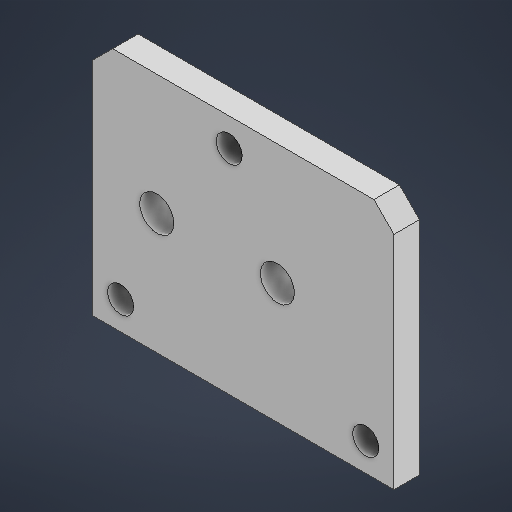
# Autodesk Inventor part: PlacaRedutor
Saved by Autodesk Inventor 2027 (Build 310192060, 192F)
## iProperties
Created: 2026-09-10
Part Number: PlacaRedutor
Material: Genérico
Document SubType Name: Modeling
Designer: Giovanna Oliveira
Density: 1 g/cm^3
Appearance: Padrão
Author: Giovanna Oliveira
Autodesk Inventor part; units mm, degrees
ref_plane "YZ Plane" through (0, 0, 0) normal (1, 0, 0) x (0, 1, 0)
ref_plane "XZ Plane" through (0, 0, 0) normal (0, 1, 0) x (-1, 0, 0)
ref_plane "XY Plane" through (0, 0, 0) normal (0, 0, 1) x (1, 0, 0)
sketch "Esboço5" plane through (0, 0, 0) normal (0, 0, 1) x (1, 0, 0)
  line L0 (-65, 60) -> (65, 60)
  line L1 (75, 50) -> (75, -60)
  line L2 (75, -60) -> (-75, -60)
  line L3 (-75, -60) -> (-75, 50)
  line L4 (-75, 60) -> (75, -60) construction
  line L5 (75, 60) -> (-75, -60) construction
  line L6 (-75, -60) -> (-61, -60) construction
  line L7 (-61, -60) -> (-61, -46) construction
  line L8 (-61, -46) -> (-75, -46) construction
  line L9 (-75, -46) -> (-75, -60) construction
  line L10 (75, -60) -> (61, -60) construction
  line L11 (61, -60) -> (61, -46) construction
  line L12 (61, -46) -> (75, -46) construction
  line L13 (75, -46) -> (75, -60) construction
  line L14 (-75, 28.5121) -> (-7, 28.5121) construction
  line L15 (-7, 60) -> (-7, 46) construction
  line L16 (-7, 0) -> (-7, -60) construction
  line L17 (-75, -11.3591) -> (-43, -11.3591) construction
  line L18 (-43, -11.3591) -> (17, -11.3591) construction
  circle A0 centre (-7, 46) radius 6.5
  circle A1 centre (-61, -46) radius 6.5
  circle A2 centre (61, -46) radius 6.5
  circle A3 centre (-43, 0) radius 8.5
  circle A4 centre (17, 0) radius 8.5
  line L19 (-65, 60) -> (-75, 50)
  line L20 (65, 60) -> (75, 50)
  point P0 (0, 0)
  dimension "d43" = 150
  dimension "d44" = 120
  dimension "d45" = 14
  dimension "d46" = 14
  dimension "d50" = 68
  dimension "d51" = 14
  dimension "d52" = 60
  dimension "d53" = 32
  dimension "d54" = 60
  dimension "d55" = 13
  dimension "d57" = 13
  dimension "d59" = 17
  dimension "d60" = 10
  dimension "d61" = 45
  constraints: 42 end point, 9 point on line, 6 parallel, 5 centre point, 5 horizontal, 3 coincident, 3 perpendicular, 2 midpoint, 1 vertical
  measures "d43" distance of L1.end L2.end
  measures "d44" distance of L5.start L1.end
  measures "d45" distance of L8.end L7.end
  measures "d46" distance of L7.end L6.end
  measures "d50" distance of L14.start L14.end
  measures "d51" distance of L15.start L15.end
  measures "d52" distance of L16.start L16.end
  measures "d53" distance of L17.start L17.end
  measures "d54" distance of L17.end L18.end
  measures "d55" diameter of A0
  measures "d57" diameter of A2
  measures "d59" diameter of A4
  measures "d60" distance of L0.start L4.start
  measures "d61" angle of L0 L19
extrude "Extrusão2" add sketch "Esboço5" against normal blind 12.7
